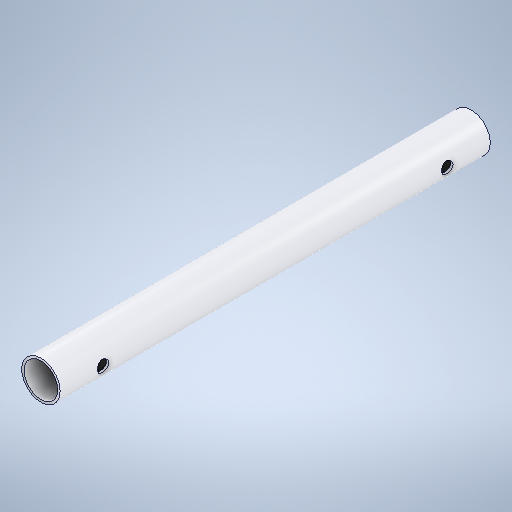
# Autodesk Inventor part: Steering PVC
Saved by Autodesk Inventor 2025.2 (Build 292293000, 293)
## iProperties
Created: 2025-02-05
Part Number: Steering PVC
Material: PVC-Piping
Document SubType Name: Modeling
Designer: eason
Density: 1.4 g/cm^3
Appearance: PTFE
Author: eason
Autodesk Inventor part; units mm, degrees
ref_plane "XZ Plane" through (0, 0, 0) normal (0, 1, 0) x (-1, 0, 0)
ref_plane "XY Plane" through (0, 0, 0) normal (0, 0, 1) x (1, 0, 0)
sketch "Sketch1" plane through (0, 0, 0) normal (0, 0, 1) x (1, 0, 0)
  circle A0 centre (0, 0) radius 13.4
  circle A1 centre (0, 0) radius 11.75
  dimension "d0" = 26.8
  dimension "d3" = 23.5
  constraints: 2 centre point, 2 coincident
  measures "d0" diameter of A0
  measures "d3" diameter of A1
extrude "Extrusion1" add sketch "Sketch1" along normal blind 300
ref_plane "Work Plane1" through (13.4, 0, 0) normal (1, 0, 0) x (0, 1, 0)
sketch "Sketch2" plane through (13.4, 0, 0) normal (1, 0, 0) x (0, 1, 0)
  circle A0 centre (0, 30) radius 4
  line L0 (0, -60) -> (0, 360) projected
  line L1 (13.4, 0) -> (-13.4, 0) projected
  circle A1 centre (0, 270) radius 4
  line L2 (13.4, 300) -> (-13.4, 300) projected
  point P0 (0, 0)
  dimension "d4" = 8
  dimension "d5" = 30
  dimension "d6" = 8
  dimension "d7" = 30
  constraints: 2 centre point, 2 point on line
  measures "d4" diameter of A0
  measures "d5" distance from line of L1 A0.centre
  measures "d6" diameter of A1
  measures "d7" distance from line of L2 A1.centre
extrude "Extrusion2" cut sketch "Sketch2" against normal through all
equation "\"d0\" = PVC_out"
equation "\"d3\" = PVC_in"
equation "\"PVC_out\" = 26.8"
equation "\"PVC_in\" = 23.5"
body "Solid1"
